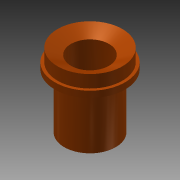
# Autodesk Inventor part: Phenolic
Saved by Autodesk Inventor 2015 (Build 190159000, 159)
## iProperties
Created: 2016-01-09
Part Number: Phenolic
Material: Phenolic Resin
Document SubType Name: Modeling
Designer: Jared
Density: 1.38 g/cm^3
Appearance: Smooth - Light Orange
Author: Jared
Autodesk Inventor part; units mm, degrees
ref_plane "YZ Plane" through (0, 0, 0) normal (1, 0, 0) x (0, 1, 0)
ref_plane "XZ Plane" through (0, 0, 0) normal (0, 1, 0) x (-1, 0, 0)
ref_plane "XY Plane" through (0, 0, 0) normal (0, 0, 1) x (1, 0, 0)
sketch "Sketch1" plane through (0, 0, 0) normal (0, 0, 1) x (1, 0, 0)
  arc A0 (-19.4827, -3.287) -> (-19.05, 0) centre (-31.75, 0) ccw
  line L0 (-19.4827, -3.287) -> (-58.7375, -149.7878)
  line L1 (-65.8876, 46.8376) -> (-65.8876, 21.4376)
  line L2 (-65.8876, 21.4376) -> (-71.4375, 21.4376)
  line L3 (-44.45, 34.1376) -> (-38.6524, 34.1376)
  line L4 (-44.45, 34.1376) -> (0, 34.1376) construction
  line L5 (-37.3992, -46.4536) -> (-31.0492, -46.4536)
  line L6 (-71.4375, 21.4376) -> (-71.4375, 8.7376)
  line L7 (-71.4375, 8.7376) -> (-58.7375, 8.7376)
  line L8 (-58.7375, 8.7376) -> (-52.3875, 8.7376)
  line L9 (-52.3875, 8.7376) -> (-52.3875, -102.3907)
  line L10 (-71.4375, 8.7376) -> (-71.4375, -0.7874)
  line L11 (-71.4375, 8.7376) -> (-61.9125, 8.7376) construction
  line L12 (-71.4375, -0.7874) -> (-58.7375, -0.7874)
  line L13 (-58.7375, -0.7874) -> (-58.7375, -51.5874)
  line L14 (-58.7375, -51.5874) -> (-71.4375, -51.5874)
  line L15 (-71.4375, -0.7874) -> (-65.0875, -0.7874)
  line L16 (-65.0875, -0.7874) -> (-65.0875, -6.731)
  line L17 (-65.0875, -6.731) -> (-71.4375, -6.731)
  line L18 (-71.4375, 21.4376) -> (-71.4375, -0.7874)
  line L19 (-71.4375, -6.731) -> (-71.4375, -51.5874)
  line L20 (-58.7375, -51.5874) -> (-58.7375, -126.0892)
  line L21 (-58.7375, -51.5874) -> (0, -51.5874) construction
  line L22 (-46.0375, -102.3907) -> (-52.3875, -102.3907)
  line L23 (-65.0875, -51.5907) -> (-58.7375, -51.5907)
  line L24 (-58.7375, -149.7878) -> (-61.9125, -161.637)
  line L25 (-58.7375, -149.7878) -> (-34.203, -149.7878) construction
  line L26 (-65.0875, -161.637) -> (-61.9125, -161.637)
  line L27 (-58.7375, -126.0892) -> (-52.3875, -126.0892)
  line L28 (0, 34.1376) -> (0, 0)
  line L29 (-65.0875, -100.6892) -> (-65.0875, -161.637)
  line L30 (-58.7375, -51.5907) -> (-61.9125, -51.5907)
  line L31 (-65.0875, -100.6892) -> (-58.7375, -100.6892)
  line L32 (-65.8876, 46.8376) -> (-18.3062, 46.8376) construction
  line L33 (-65.8876, 46.8376) -> (-14.7047, 46.8376) construction
  line L34 (-65.8876, 46.8376) -> (-33.5957, 31.7796)
  line L35 (-65.8876, 46.8376) -> (-30.2574, 46.8376) construction
  arc A1 (-19.05, 0) -> (-33.5957, 31.7796) centre (-61.0391, 0) ccw
  line L36 (-44.45, 34.1376) -> (-44.45, -46.4536)
  line L37 (-44.45, 34.1376) -> (36.1412, 34.1376) construction
  line L38 (-44.45, -46.4536) -> (-37.3992, -46.4536)
  dimension "d86" = 19.05
  dimension "d87" = 25.4
  dimension "d88" = 5.5499
  dimension "d89" = 65.8876
  dimension "d90" = 12.7
  dimension "d91" = 12.7
  dimension "d92" = 44.45
  dimension "d93" = 6.35
  dimension "d94" = 105
  dimension "d95" = 12.7
  dimension "d96" = 12.7
  dimension "d97" = 6.35
  dimension "d98" = 9.525
  dimension "d99" = 50.8
  dimension "d100" = 12.7
  dimension "d101" = 6.35
  dimension "d102" = 5.9436
  dimension "d103" = 6.35
  dimension "d104" = 50.8
  dimension "d105" = 6.35
  dimension "d106" = 105
  dimension "d107" = 3.175
  dimension "d108" = 6.35
  dimension "d109" = 60.9478
  dimension "d110" = 3.175
  dimension "d111" = 6.35
  dimension "d112" = 25.4
  dimension "d113" = 25
  dimension "d114" = 41.9891
  dimension "d115" = 32.2919
  dimension "d116" = 90
  dimension "d117" = 80.5912
  constraints: 79 end point, 15 perpendicular, 13 horizontal, 8 point on line, 4 point on circle, 4 vertical, 3 equal length, 3 horizontal alignment, 2 centre point, 2 collinear, 2 midpoint, 1 parallel, 1 tangent, 1 vertical alignment, 1 other
  measures "d86" distance of A1.start L28.end
  measures "d87" distance of L1.start L1.end
  measures "d88" distance of L1.end L6.start
  measures "d89" distance from line of L28.end L1
  measures "d90" vertical distance of L3.start L1.start
  measures "d91" radius of A0
  measures "d92" horizontal distance of L28.end L3.start
  measures "d93" distance of L5.start L5.end
  measures "d94" angle of L5 L0
  measures "d95" distance of L6.start L6.end
  measures "d96" distance of L6.end L8.start
  measures "d97" distance of L8.start L9.start
  measures "d98" distance of L6.end L18.end
  measures "d99" distance of L12.end L21.start
  measures "d100" distance of L18.end L12.end
  measures "d101" distance of L18.end L15.end
  measures "d102" distance of L15.end L17.start
  measures "d103" distance of L9.end L22.start
  measures "d104" distance between parallel lines of L22 L23
  measures "d105" distance of L23.start L30.start
  measures "d106" angle of L24 L25
  measures "d107" distance of L24.end L29.end
  measures "d108" distance of L20.end L27.end
  measures "d109" distance of L31.start L29.end
  measures "d110" distance of L30.start L30.end
  measures "d111" distance from line of L20 L31.start
  measures "d112" distance between parallel lines of L31 L27
  measures "d113" angle of L34 L35
  measures "d114" radius of A1
  measures "d115" horizontal distance of L1.start L34.end
  measures "d116" angle of L36 L37
  measures "d117" distance of L3.start L38.start
revolve "Revolution1" add sketch "Sketch1" angle 360 about axis through (0, 34.1376, 0) along (0, -1, 0) contours L0 L22 L9 L8 L7 L6 L2 L1 L34 L3 L36 L38 L5
body "Solid1"
